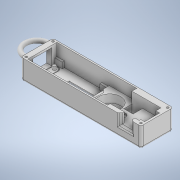
# Autodesk Inventor part: RespiraCheck-Enclosure-Top
Saved by Autodesk Inventor 2022 (Build 260153000, 153)
## iProperties
Created: 2022-04-28
Part Number: RespiraCheck-Enclosure-Top
Material: Generic
Document SubType Name: Modeling
Designer: incep
Density: 1 g/cm^3
Appearance: Default
Author: incep
## iProperties of the stored document RespiraCheck-Enclosure-Top_3DPrint.ipt
Created: 2022-04-28
Part Number: RespiraCheck-Enclosure-Top_3DPrint
Material: Generic
Document SubType Name: Modeling
Designer: incep
Density: 1 g/cm^3
Appearance: Default
Author: incep
Autodesk Inventor part; units mm, degrees
ref_plane "YZ Plane" through (0, 0, 0) normal (1, 0, 0) x (0, 1, 0)
ref_plane "XZ Plane" through (0, 0, 0) normal (0, 1, 0) x (-1, 0, 0)
sketch "Sketch1" plane through (0, 0, 0) normal (0, 1, 0) x (-1, 0, 0)
  line L0 (56, 15) -> (-56, 15)
  line L1 (-56, 15) -> (-56, -15)
  line L2 (-56, -15) -> (56, -15)
  line L3 (56, -15) -> (56, 15)
  point P0 (0, 0)
  point P1 (-56, 0)
  point P2 (0, -15)
  dimension "d0" = 30
  dimension "d1" = 112
  constraints: 8 end point, 2 midpoint, 2 parallel, 1 horizontal, 1 horizontal alignment, 1 perpendicular, 1 vertical alignment
  measures "d0" distance of L2.end L0.start
  measures "d1" distance of L1.end L2.end
extrude "Extrusion1" add sketch "Sketch1" along normal blind 19
sketch "Sketch2" plane through (0, 19, 0) normal (0, 1, 0) x (1, 0, 0)
  circle A0 centre (-53.5, 12.5) radius 2.5 construction
  line L0 (56, 15) -> (-56, 15) construction
  line L1 (-56, 15) -> (-56, -15) construction
  circle A1 centre (-53.5, -12.5) radius 2.5 construction
  circle A2 centre (53.5, 12.5) radius 2.5 construction
  circle A3 centre (53.5, -12.5) radius 2.5 construction
  line L2 (-56, -15) -> (56, -15) construction
  line L3 (56, -15) -> (56, 15) construction
  line L4 (-51, 13.6) -> (-2, 13.6)
  line L5 (-2, -13.6) -> (-51, -13.6)
  line L6 (-51, -13.6) -> (-51, 13.6)
  line L7 (-2, 8) -> (1, 8)
  line L8 (1, 8) -> (1, -8)
  line L9 (1, -8) -> (-2, -8)
  line L10 (-2, -8) -> (-2, 8) construction
  line L11 (-2, 8) -> (1, 5)
  line L12 (-2, -8) -> (1, -5)
  line L13 (-2, 13.6) -> (-2, 8)
  line L14 (-2, -8) -> (-2, -13.6)
  circle A4 centre (-53.5, 12.5) radius 1
  circle A5 centre (-53.5, -12.5) radius 1
  circle A6 centre (53.5, 12.5) radius 1
  circle A7 centre (53.5, -12.5) radius 1
  point P0 (0, 0)
  point P1 (-2, 0)
  point P2 (1, 0)
  point P3 (-51, 0)
  dimension "d4" = 5
  dimension "d5" = 5
  dimension "d6" = 5
  dimension "d7" = 5
  dimension "d8" = 27.2
  dimension "d10" = 3
  dimension "d11" = 16
  dimension "d14" = 49
  dimension "d15" = 45
  dimension "d16" = 45
  dimension "d64" = 2
  dimension "d65" = 2
  dimension "d66" = 2
  dimension "d67" = 2
  constraints: 22 end point, 9 tangent, 8 centre point, 5 parallel, 4 coincident, 3 perpendicular, 2 collinear, 2 horizontal, 2 horizontal alignment, 2 midpoint, 2 point on line
  measures "d4" diameter of A0
  measures "d5" diameter of A1
  measures "d6" diameter of A2
  measures "d7" diameter of A3
  measures "d8" distance of L5.end L4.start
  measures "d10" distance of L7.start L7.end
  measures "d11" distance of L7.end L8.end
  measures "d14" distance between parallel lines of L6 L13
  measures "d15" angle of L7 L11
  measures "d16" angle of L9 L12
  measures "d64" diameter of A4
  measures "d65" diameter of A5
  measures "d66" diameter of A6
  measures "d67" diameter of A7
extrude "Extrusion2" cut sketch "Sketch2" against normal blind 11.5 contours L4 L13 L11 L8 L12 L14 L5 L6 | A4 | A5 | A6 | A7
sketch "Sketch3" plane through (0, 7.5, 0) normal (0, 1, 0) x (1, 0, 0)
  line L0 (-2, 11.6) -> (-2, -11.6)
  line L1 (-51, -11.6) -> (-51, 11.6)
  line L2 (-51, -13.6) -> (-51, 13.6) projected
  line L3 (-2, 13.6) -> (-2, 8) projected
  line L4 (-9, -11.6) -> (-9, -13.6)
  line L5 (-9, -13.6) -> (-44, -13.6)
  line L6 (-44, -13.6) -> (-44, -11.6)
  line L7 (-2, -8) -> (-2, -13.6) projected
  line L8 (-2, -11.6) -> (-9, -11.6)
  line L9 (-44, -11.6) -> (-51, -11.6)
  line L10 (-51, 11.6) -> (-44, 11.6)
  line L11 (-9, 11.6) -> (-2, 11.6)
  line L12 (-51, 13.6) -> (-2, 13.6) projected
  line L13 (-9, 11.6) -> (-9, 13.6)
  line L14 (-9, 13.6) -> (-44, 13.6)
  line L15 (-44, 13.6) -> (-44, 11.6)
  line L16 (-2, -13.6) -> (-51, -13.6) projected
  point P0 (0, 0)
  point P1 (-2, 0)
  point P2 (-8.9823, 10)
  point P3 (-44, 13.6)
  dimension "d20" = 7
  dimension "d21" = 7
  dimension "d93" = 2
  dimension "d94" = 2
  dimension "d95" = 2
  constraints: 24 end point, 7 parallel, 4 collinear, 3 point on line, 2 horizontal, 2 perpendicular, 1 horizontal alignment, 1 midpoint, 1 vertical
  measures "d20" distance between parallel lines of L4 L7
  measures "d21" distance between parallel lines of L2 L6
  measures "d93" distance of L14.end L10.end
  measures "d94" distance of L11.start L13.end
  measures "d95" distance of L5.end L6.end
extrude "Extrusion3" cut sketch "Sketch3" against normal blind 5.5 contours L0 L8 L4 L5 L6 L9 L1 L10 L15 L12 L13 L11
sketch "Sketch4" plane through (0, 2, 0) normal (0, 1, 0) x (1, 0, 0)
  line L0 (-31, 5.1) -> (-7, 5.1)
  line L1 (-7, 5.1) -> (-7, -8.9)
  line L2 (-7, -8.9) -> (-31, -8.9)
  line L3 (-31, -8.9) -> (-31, 5.1)
  line L4 (-2, 8) -> (-2, -8) projected
  line L5 (-51, 13.6) -> (-2, 13.6) projected
  line L6 (-2, -13.6) -> (-51, -13.6) projected
  point P0 (0, 0)
  dimension "d24" = 5
  dimension "d25" = 8.5
  dimension "d26" = 4.7
  dimension "d27" = 24
  constraints: 8 end point, 2 parallel, 1 horizontal, 1 perpendicular
  measures "d24" distance between parallel lines of L4 L1
  measures "d25" distance between parallel lines of L0 L5
  measures "d26" distance between parallel lines of L6 L2
  measures "d27" distance between parallel lines of L3 L1
extrude "Extrusion4" cut sketch "Sketch4" against normal blind 2
sketch "Sketch5" plane through (0, 19, 0) normal (0, 1, 0) x (1, 0, 0)
  line L0 (-51, 13.6) -> (-2, 13.6) projected
  line L1 (-2, 13.6) -> (23.5, 13.6)
  line L2 (23.5, 13.6) -> (23.5, -13.6)
  line L3 (23.5, -13.6) -> (-2, -13.6)
  line L4 (-2, -13.6) -> (-2, 13.6)
  circle A0 centre (53.5, 12.5) radius 2.5 construction
  circle A1 centre (53.5, -12.5) radius 2.5 construction
  line L5 (-2, -13.6) -> (-51, -13.6) projected
  line L6 (1, 5) -> (1, -5) projected
  point P0 (0, 0)
  dimension "d43" = 22.5
  constraints: 8 end point, 2 parallel, 1 collinear, 1 horizontal, 1 perpendicular
  measures "d43" distance between parallel lines of L2 L6
extrude "Extrusion5" cut sketch "Sketch5" against normal blind 10.5
sketch "Sketch6" plane through (0, 8.5, 0) normal (0, 1, 0) x (1, 0, 0)
  circle A0 centre (12, 0) radius 10.1
  line L0 (1, -5) -> (1, 5) projected
  point P0 (0, 0)
  dimension "d32" = 20.2
  dimension "d33" = 11
  constraints: 1 centre point, 1 horizontal alignment
  measures "d32" diameter of A0
  measures "d33" distance from line of L0 A0.centre
extrude "Extrusion6" cut sketch "Sketch6" against normal blind 7.5
sketch "Sketch7" plane through (12, 1, 0) normal (0, 1, 0) x (1, 0, 0)
  circle A0 centre (0, 0) radius 10.1 projected
  circle A1 centre (0, 0) radius 6.5
  point P0 (-12, 0)
  dimension "d36" = 13
  constraints: 1 centre point, 1 coincident
  measures "d36" diameter of A1
extrude "Extrusion7" cut sketch "Sketch7" against normal blind 2 contours A1
sketch "Sketch8" plane through (0, 19, 0) normal (0, 1, 0) x (1, 0, 0)
  line L0 (23.5, 9.15) -> (50.6, 9.15)
  line L1 (50.6, 9.15) -> (50.6, -11.15)
  line L2 (50.6, -11.15) -> (23.5, -11.15)
  line L3 (23.5, -11.15) -> (23.5, 9.15)
  circle A0 centre (12, 0) radius 10.1 projected
  line L4 (23.5, -1) -> (50.6, -1) construction
  line L5 (23.5, 13.6) -> (23.5, -13.6) projected
  line L6 (50.6, 4.35) -> (54.1, 4.35)
  line L7 (54.1, 4.35) -> (54.1, -9.65)
  line L8 (54.1, -9.65) -> (50.6, -9.65)
  line L9 (50.6, -9.65) -> (50.6, 4.35)
  point P0 (0, 0)
  point P1 (50.6, 4.35)
  point P2 (50.6, -9.65)
  dimension "d39" = 20.3
  dimension "d42" = 1
  dimension "d46" = 27.1
  dimension "d47" = 14
  dimension "d48" = 3.5
  dimension "d49" = 1.5
  constraints: 18 end point, 4 parallel, 2 collinear, 2 horizontal, 2 midpoint, 2 perpendicular
  measures "d39" distance of L2.end L0.start
  measures "d42" vertical distance of L4.start A0.centre
  measures "d46" distance between parallel lines of L1 L3
  measures "d47" distance of L6.end L7.end
  measures "d48" distance of L6.start L6.end
  measures "d49" distance from line of L1.end L8
extrude "Extrusion8" cut sketch "Sketch8" against normal blind 9 contours L0 L1 L2 L3 | L6 L7 L8 L1
sketch "Sketch9" plane through (0, 10, 0) normal (0, 1, 0) x (1, 0, 0)
  line L0 (23.5, 9.15) -> (33.5, 9.15)
  line L1 (33.5, 9.15) -> (33.5, 0.15)
  line L2 (33.5, 0.15) -> (23.5, 0.15)
  line L3 (23.5, 0.15) -> (23.5, 9.15)
  line L4 (23.5, 9.15) -> (50.6, 9.15) projected
  line L5 (23.5, -11.15) -> (23.5, 9.15) projected
  point P0 (0, 0)
  dimension "d50" = 10
  dimension "d51" = 9
  constraints: 8 end point, 2 collinear, 2 parallel, 1 horizontal, 1 perpendicular
  measures "d50" distance of L1.end L2.end
  measures "d51" distance of L0.end L1.end
extrude "Extrusion9" cut sketch "Sketch9" against normal blind 10.5
sketch "Sketch10" plane through (50.6, 19, 11.15) normal (0, 0, -1) x (-1, 0, 0)
  line L0 (4, 0) -> (14, 0)
  line L1 (14, 0) -> (14, -9)
  line L2 (14, -9) -> (4, -9)
  line L3 (4, -9) -> (4, 0)
  line L4 (0, 0) -> (0, -9) projected
  line L5 (0, 0) -> (27.1, 0) projected
  line L6 (0, -9) -> (27.1, -9) projected
  point P0 (50.6, -19)
  dimension "d54" = 4
  dimension "d55" = 10
  constraints: 8 end point, 2 collinear, 2 parallel, 1 horizontal, 1 perpendicular
  measures "d54" distance between parallel lines of L4 L3
  measures "d55" distance between parallel lines of L1 L3
extrude "Extrusion10" cut sketch "Sketch10" against normal through all contours L0 L1 L2 L3
sketch "Sketch11" plane through (-56, 0, -15) normal (-1, 0, 0) x (0, 0, 1)
  line L0 (6, 17) -> (24, 17)
  line L1 (24, 17) -> (24, 2)
  line L2 (24, 2) -> (6, 2)
  line L3 (6, 2) -> (6, 17)
  line L4 (30, 0) -> (30, 19) projected
  line L5 (0, 0) -> (0, 19) projected
  line L6 (0, 0) -> (30, 0) projected
  line L7 (0, 19) -> (30, 19) projected
  point P0 (15, 0)
  dimension "d58" = 6
  dimension "d59" = 6
  dimension "d60" = 2
  dimension "d61" = 2
  constraints: 8 end point, 2 parallel, 1 horizontal, 1 perpendicular
  measures "d58" distance between parallel lines of L4 L1
  measures "d59" distance between parallel lines of L5 L3
  measures "d60" distance between parallel lines of L6 L2
  measures "d61" distance between parallel lines of L7 L0
extrude "Extrusion11" cut sketch "Sketch11" against normal up to surface (5 mm away) contours L0 L1 L2 L3
sketch "Sketch12" plane through (0, 0, 0) normal (0, -1, 0) x (1, 0, 0)
  line L0 (-39.2331, -12.5927) -> (-39.2331, 29.3378) construction
  line L1 (-39.2331, 29.3378) -> (-35.2988, 29.3378) construction
  line L2 (-35.2988, 29.3378) -> (-35.2988, -12.5927) construction
  line L3 (-35.2988, -12.5927) -> (-39.2331, -12.5927) construction
  line L4 (-36.3768, -10.4806) -> (-37.3923, -11.2247)
  spline S0 degree 2 poles (-37.3923, -11.2247) (-37.4874, -10.8555) (-37.9238, -10.5058) (-38.2455, -10.5058) knots 0 0 0 1 2 2 2
  spline S1 degree 2 poles (-38.2455, -10.5058) (-38.4554, -10.5058) (-38.8023, -10.654) (-38.9226, -10.7967) knots 0 0 0 1 2 2 2
  spline S2 degree 2 poles (-38.9226, -10.7967) (-39.0345, -10.9254) (-39.1268, -11.2723) (-39.1268, -11.5465) knots 0 0 0 1 2 2 2
  line L5 (-39.1268, -11.5465) -> (-39.1268, -12.3382)
  line L6 (-39.1268, -12.3382) -> (-36.3768, -12.3382)
  line L7 (-36.3768, -12.3382) -> (-36.3768, -11.829)
  line L8 (-36.3768, -11.829) -> (-37.4315, -11.829)
  line L9 (-37.4315, -11.829) -> (-36.3768, -11.11)
  line L10 (-36.3768, -11.11) -> (-36.3768, -10.4806)
  spline S3 degree 2 poles (-38.2316, -11.0205) (-38.0133, -11.0177) (-37.8119, -11.2863) (-37.8147, -11.58) knots 0 0 0 1 2 2 2
  line L11 (-37.8147, -11.58) -> (-37.8147, -11.829)
  line L12 (-37.8147, -11.829) -> (-38.64, -11.829)
  line L13 (-38.64, -11.829) -> (-38.64, -11.6024)
  spline S4 degree 2 poles (-38.64, -11.6024) (-38.64, -11.3646) (-38.5365, -11.11) (-38.3546, -11.0177) (-38.2316, -11.0205) knots 0 0 0 1 2 3 3 3
  spline S5 degree 2 poles (-37.3783, -8.1726) (-37.7, -8.1754) (-38.198, -8.4496) (-38.4833, -8.9279) (-38.4861, -9.2385) knots 0 0 0 1 2 3 3 3
  spline S6 degree 2 poles (-38.4861, -9.2385) (-38.4833, -9.5434) (-38.1952, -10.033) (-37.7084, -10.3211) (-37.4007, -10.3239) knots 0 0 0 1 2 3 3 3
  spline S7 degree 2 poles (-37.4007, -10.3239) (-37.0957, -10.3211) (-36.6146, -10.0274) (-36.332, -9.5266) (-36.3292, -9.2077) knots 0 0 0 1 2 3 3 3
  spline S8 degree 2 poles (-36.3292, -9.2077) (-36.3292, -8.9979) (-36.4803, -8.6006) (-36.774, -8.2985) (-36.9866, -8.2258) knots 0 0 0 1 2 3 3 3
  line L14 (-36.9866, -8.2258) -> (-36.9866, -8.7657)
  spline S9 degree 2 poles (-36.9866, -8.7657) (-36.8775, -8.858) (-36.7824, -9.0678) (-36.7824, -9.2189) knots 0 0 0 1 2 2 2
  spline S10 degree 2 poles (-36.7824, -9.2189) (-36.7852, -9.4427) (-37.0006, -9.742) (-37.1881, -9.7896) knots 0 0 0 1 2 2 2
  line L15 (-37.1881, -9.7896) -> (-37.1881, -8.1922)
  spline S11 degree 2 poles (-37.1881, -8.1922) (-37.2384, -8.181) (-37.3251, -8.1726) (-37.3783, -8.1726) knots 0 0 0 1 2 2 2
  line L16 (-37.6245, -8.6622) -> (-37.6245, -9.8036)
  spline S12 degree 2 poles (-37.6245, -9.8036) (-37.8231, -9.7448) (-38.0329, -9.4511) (-38.0329, -9.2301) knots 0 0 0 1 2 2 2
  spline S13 degree 2 poles (-38.0329, -9.2301) (-38.0329, -9.0007) (-37.8231, -8.7097) (-37.6245, -8.6622) knots 0 0 0 1 2 2 2
  spline S14 degree 2 poles (-37.0314, -6.4913) (-37.258, -6.4857) (-37.5378, -6.7458) (-37.6357, -7.0648) knots 0 0 0 1 2 2 2
  spline S15 degree 2 poles (-37.6357, -7.0648) (-37.686, -7.2298) (-37.7476, -7.3809) (-37.8063, -7.4173) (-37.8595, -7.4145) knots 0 0 0 1 2 3 3 3
  spline S16 degree 2 poles (-37.8595, -7.4145) (-37.935, -7.4117) (-38.0329, -7.3082) (-38.0329, -7.2242) knots 0 0 0 1 2 2 2
  spline S17 degree 2 poles (-38.0329, -7.2242) (-38.0329, -7.1459) (-37.949, -7.048) (-37.8707, -7.0312) knots 0 0 0 1 2 2 2
  line L17 (-37.8707, -7.0312) -> (-37.8707, -6.5472)
  spline S18 degree 2 poles (-37.8707, -6.5472) (-38.0637, -6.5584) (-38.3379, -6.7486) (-38.4861, -7.048) (-38.4861, -7.2242) knots 0 0 0 1 2 3 3 3
  spline S19 degree 2 poles (-38.4861, -7.2242) (-38.4805, -7.518) (-38.128, -7.9012) (-37.8595, -7.9096) knots 0 0 0 1 2 2 2
  spline S20 degree 2 poles (-37.8595, -7.9096) (-37.6357, -7.9124) (-37.3475, -7.6411) (-37.2468, -7.3361) knots 0 0 0 1 2 2 2
  spline S21 degree 2 poles (-37.2468, -7.3361) (-37.1937, -7.1739) (-37.1181, -7.0228) (-37.0426, -6.9836) (-36.9838, -6.9864) knots 0 0 0 1 2 3 3 3
  spline S22 degree 2 poles (-36.9838, -6.9864) (-36.8943, -6.9892) (-36.7852, -7.1123) (-36.7824, -7.2102) knots 0 0 0 1 2 2 2
  spline S23 degree 2 poles (-36.7824, -7.2102) (-36.7824, -7.3165) (-36.8999, -7.4508) (-37.0314, -7.4844) knots 0 0 0 1 2 2 2
  line L18 (-37.0314, -7.4844) -> (-37.0314, -7.9852)
  spline S24 degree 2 poles (-37.0314, -7.9852) (-36.6733, -7.9404) (-36.3292, -7.5403) (-36.3292, -7.227) knots 0 0 0 1 2 2 2
  spline S25 degree 2 poles (-36.3292, -7.227) (-36.332, -7.02) (-36.5167, -6.6871) (-36.8328, -6.4941) (-37.0314, -6.4913) knots 0 0 0 1 2 3 3 3
  spline S26 degree 2 poles (-37.4147, -4.0602) (-37.728, -4.063) (-38.2092, -4.326) (-38.4833, -4.7876) (-38.4861, -5.0869) knots 0 0 0 1 2 3 3 3
  spline S27 degree 2 poles (-38.4861, -5.0869) (-38.4861, -5.2967) (-38.3351, -5.6436) (-38.1952, -5.7639) knots 0 0 0 1 2 2 2
  line L19 (-38.1952, -5.7639) -> (-38.4386, -5.7639)
  line L20 (-38.4386, -5.7639) -> (-38.4386, -6.2171)
  line L21 (-38.4386, -6.2171) -> (-35.6886, -6.2171)
  line L22 (-35.6886, -6.2171) -> (-35.6886, -5.7219)
  line L23 (-35.6886, -5.7219) -> (-36.5698, -5.7219)
  spline S28 degree 2 poles (-36.5698, -5.7219) (-36.4467, -5.5849) (-36.3292, -5.2771) (-36.3292, -5.0897) knots 0 0 0 1 2 2 2
  spline S29 degree 2 poles (-36.3292, -5.0897) (-36.332, -4.7903) (-36.6118, -4.326) (-37.0985, -4.063) (-37.4147, -4.0602) knots 0 0 0 1 2 3 3 3
  spline S30 degree 2 poles (-37.4035, -4.5582) (-37.1349, -4.5637) (-36.788, -4.8911) (-36.7824, -5.1428) knots 0 0 0 1 2 2 2
  spline S31 degree 2 poles (-36.7824, -5.1428) (-36.788, -5.4086) (-37.1349, -5.7471) (-37.4119, -5.7527) knots 0 0 0 1 2 2 2
  spline S32 degree 2 poles (-37.4119, -5.7527) (-37.6832, -5.7471) (-38.0273, -5.4114) (-38.0329, -5.1484) knots 0 0 0 1 2 2 2
  spline S33 degree 2 poles (-38.0329, -5.1484) (-38.0273, -4.8939) (-37.6776, -4.5637) (-37.4035, -4.5582) knots 0 0 0 1 2 2 2
  line L24 (-36.3768, -3.2657) -> (-38.4386, -3.2657)
  line L25 (-38.4386, -3.2657) -> (-38.4386, -3.7608)
  line L26 (-38.4386, -3.7608) -> (-36.3768, -3.7608)
  line L27 (-36.3768, -3.7608) -> (-36.3768, -3.2657)
  line L28 (-38.7351, -3.2629) -> (-39.2303, -3.2629)
  line L29 (-39.2303, -3.2629) -> (-39.2303, -3.758)
  line L30 (-39.2303, -3.758) -> (-38.7351, -3.758)
  line L31 (-38.7351, -3.758) -> (-38.7351, -3.2629)
  line L32 (-38.0105, -1.9312) -> (-38.4861, -1.9312)
  line L33 (-38.4861, -1.9312) -> (-38.4861, -1.9676)
  spline S34 degree 2 poles (-38.4861, -1.9676) (-38.4889, -2.1215) (-38.377, -2.3201) (-38.2372, -2.4152) knots 0 0 0 1 2 2 2
  line L34 (-38.2372, -2.4152) -> (-38.4386, -2.4152)
  line L35 (-38.4386, -2.4152) -> (-38.4386, -2.8684)
  line L36 (-38.4386, -2.8684) -> (-36.3768, -2.8684)
  line L37 (-36.3768, -2.8684) -> (-36.3768, -2.3733)
  line L38 (-36.3768, -2.3733) -> (-37.5238, -2.3733)
  spline S35 degree 2 poles (-37.5238, -2.3733) (-37.7616, -2.3733) (-38.005, -2.155) (-38.0105, -1.9312) knots 0 0 0 1 2 2 2
  line L39 (-36.3768, 0.4103) -> (-38.4386, 0.4103)
  line L40 (-38.4386, 0.4103) -> (-38.4386, -0.0457)
  line L41 (-38.4386, -0.0457) -> (-38.1616, -0.0457)
  spline S36 degree 2 poles (-38.1616, -0.0457) (-38.3323, -0.1716) (-38.4861, -0.4961) (-38.4861, -0.7171) knots 0 0 0 1 2 2 2
  spline S37 degree 2 poles (-38.4861, -0.7171) (-38.4833, -1.0248) (-38.2064, -1.4948) (-37.7168, -1.7634) (-37.4007, -1.7662) knots 0 0 0 1 2 3 3 3
  spline S38 degree 2 poles (-37.4007, -1.7662) (-37.0874, -1.7634) (-36.6062, -1.4976) (-36.332, -1.0332) (-36.3292, -0.7283) knots 0 0 0 1 2 3 3 3
  spline S39 degree 2 poles (-36.3292, -0.7283) (-36.3292, -0.5129) (-36.4803, -0.1884) (-36.6453, -0.0457) knots 0 0 0 1 2 2 2
  line L42 (-36.6453, -0.0457) -> (-36.3768, -0.0457)
  line L43 (-36.3768, -0.0457) -> (-36.3768, 0.4103)
  spline S40 degree 2 poles (-37.3923, -0.0597) (-37.1293, -0.0625) (-36.788, -0.373) (-36.7824, -0.6584) knots 0 0 0 1 2 2 2
  spline S41 degree 2 poles (-36.7824, -0.6584) (-36.7852, -0.9325) (-37.1153, -1.2654) (-37.3895, -1.2682) knots 0 0 0 1 2 2 2
  spline S42 degree 2 poles (-37.3895, -1.2682) (-37.6748, -1.2626) (-38.0273, -0.9353) (-38.0329, -0.6667) knots 0 0 0 1 2 2 2
  spline S43 degree 2 poles (-38.0329, -0.6667) (-38.0273, -0.3954) (-37.6804, -0.0653) (-37.3923, -0.0597) knots 0 0 0 1 2 2 2
  line L44 (-37.1433, 3.4065) -> (-37.1433, 2.8078)
  spline S44 degree 2 poles (-37.1433, 2.8078) (-36.9699, 2.6428) (-36.8188, 2.321) (-36.8216, 2.128) knots 0 0 0 1 2 2 2
  spline S45 degree 2 poles (-36.8216, 2.128) (-36.8244, 1.8706) (-37.0762, 1.4538) (-37.4986, 1.2076) (-37.756, 1.2048) knots 0 0 0 1 2 3 3 3
  spline S46 degree 2 poles (-37.756, 1.2048) (-38.0189, 1.2076) (-38.4358, 1.4426) (-38.6792, 1.8511) (-38.682, 2.1168) knots 0 0 0 1 2 3 3 3
  spline S47 degree 2 poles (-38.682, 2.1168) (-38.6848, 2.3546) (-38.5169, 2.7015) (-38.3379, 2.8386) knots 0 0 0 1 2 2 2
  line L45 (-38.3379, 2.8386) -> (-38.3379, 3.4065)
  spline S48 degree 2 poles (-38.3379, 3.4065) (-38.7379, 3.2191) (-39.1715, 2.5337) (-39.1743, 2.1056) knots 0 0 0 1 2 2 2
  spline S49 degree 2 poles (-39.1743, 2.1056) (-39.1687, 1.7112) (-38.7911, 1.0733) (-38.1532, 0.6957) (-37.7616, 0.6901) knots 0 0 0 1 2 3 3 3
  spline S50 degree 2 poles (-37.7616, 0.6901) (-37.3615, 0.6957) (-36.7153, 1.0789) (-36.3348, 1.7308) (-36.3292, 2.1392) knots 0 0 0 1 2 3 3 3
  spline S51 degree 2 poles (-36.3292, 2.1392) (-36.3348, 2.5672) (-36.7628, 3.2386) (-37.1433, 3.4065) knots 0 0 0 1 2 2 2
  line L46 (-36.3768, 5.5075) -> (-37.5434, 5.5075)
  spline S52 degree 2 poles (-37.5434, 5.5075) (-38.0469, 5.5019) (-38.4945, 5.0738) (-38.4917, 4.699) knots 0 0 0 1 2 2 2
  spline S53 degree 2 poles (-38.4917, 4.699) (-38.4917, 4.5423) (-38.3966, 4.2849) (-38.2987, 4.1758) knots 0 0 0 1 2 2 2
  line L47 (-38.2987, 4.1758) -> (-39.1268, 4.1758)
  line L48 (-39.1268, 4.1758) -> (-39.1268, 3.6807)
  line L49 (-39.1268, 3.6807) -> (-36.3768, 3.6807)
  line L50 (-36.3768, 3.6807) -> (-36.3768, 4.1758)
  line L51 (-36.3768, 4.1758) -> (-37.4231, 4.1758)
  spline S54 degree 2 poles (-37.4231, 4.1758) (-37.7588, 4.1758) (-38.0385, 4.3968) (-38.0329, 4.6094) knots 0 0 0 1 2 2 2
  spline S55 degree 2 poles (-38.0329, 4.6094) (-38.0357, 4.8277) (-37.7504, 5.0151) (-37.4315, 5.0123) knots 0 0 0 1 2 2 2
  line L52 (-37.4315, 5.0123) -> (-36.3768, 5.0123)
  line L53 (-36.3768, 5.0123) -> (-36.3768, 5.5075)
  spline S56 degree 2 poles (-37.3783, 7.9749) (-37.7, 7.9721) (-38.198, 7.698) (-38.4833, 7.2196) (-38.4861, 6.909) knots 0 0 0 1 2 3 3 3
  spline S57 degree 2 poles (-38.4861, 6.909) (-38.4833, 6.6041) (-38.1952, 6.1145) (-37.7084, 5.8264) (-37.4007, 5.8236) knots 0 0 0 1 2 3 3 3
  spline S58 degree 2 poles (-37.4007, 5.8236) (-37.0957, 5.8264) (-36.6146, 6.1201) (-36.332, 6.6209) (-36.3292, 6.9398) knots 0 0 0 1 2 3 3 3
  spline S59 degree 2 poles (-36.3292, 6.9398) (-36.3292, 7.1496) (-36.4803, 7.5469) (-36.774, 7.849) (-36.9866, 7.9218) knots 0 0 0 1 2 3 3 3
  line L54 (-36.9866, 7.9218) -> (-36.9866, 7.3818)
  spline S60 degree 2 poles (-36.9866, 7.3818) (-36.8775, 7.2895) (-36.7824, 7.0797) (-36.7824, 6.9286) knots 0 0 0 1 2 2 2
  spline S61 degree 2 poles (-36.7824, 6.9286) (-36.7852, 6.7048) (-37.0006, 6.4055) (-37.1881, 6.3579) knots 0 0 0 1 2 2 2
  line L55 (-37.1881, 6.3579) -> (-37.1881, 7.9553)
  spline S62 degree 2 poles (-37.1881, 7.9553) (-37.2384, 7.9665) (-37.3251, 7.9749) (-37.3783, 7.9749) knots 0 0 0 1 2 2 2
  line L56 (-37.6245, 7.4853) -> (-37.6245, 6.3439)
  spline S63 degree 2 poles (-37.6245, 6.3439) (-37.8231, 6.4027) (-38.0329, 6.6964) (-38.0329, 6.9174) knots 0 0 0 1 2 2 2
  spline S64 degree 2 poles (-38.0329, 6.9174) (-38.0329, 7.1468) (-37.8231, 7.4378) (-37.6245, 7.4853) knots 0 0 0 1 2 2 2
  line L57 (-37.0538, 10.3277) -> (-37.0538, 9.7709)
  spline S65 degree 2 poles (-37.0538, 9.7709) (-36.9111, 9.6786) (-36.7824, 9.452) (-36.7824, 9.301) knots 0 0 0 1 2 2 2
  spline S66 degree 2 poles (-36.7824, 9.301) (-36.788, 9.038) (-37.1349, 8.7079) (-37.4119, 8.7023) knots 0 0 0 1 2 2 2
  spline S67 degree 2 poles (-37.4119, 8.7023) (-37.686, 8.7079) (-38.0273, 9.0296) (-38.0329, 9.2898) knots 0 0 0 1 2 2 2
  spline S68 degree 2 poles (-38.0329, 9.2898) (-38.0329, 9.4576) (-37.8931, 9.6954) (-37.7504, 9.7709) knots 0 0 0 1 2 2 2
  line L58 (-37.7504, 9.7709) -> (-37.7504, 10.3277)
  spline S69 degree 2 poles (-37.7504, 10.3277) (-38.1057, 10.2018) (-38.4833, 9.6479) (-38.4861, 9.2898) knots 0 0 0 1 2 2 2
  spline S70 degree 2 poles (-38.4861, 9.2898) (-38.4833, 8.982) (-38.2008, 8.4925) (-37.714, 8.2071) (-37.4063, 8.2043) knots 0 0 0 1 2 3 3 3
  spline S71 degree 2 poles (-37.4063, 8.2043) (-37.1041, 8.2071) (-36.6202, 8.5009) (-36.332, 8.996) (-36.3292, 9.3038) knots 0 0 0 1 2 3 3 3
  spline S72 degree 2 poles (-36.3292, 9.3038) (-36.332, 9.6674) (-36.7069, 10.1962) (-37.0538, 10.3277) knots 0 0 0 1 2 2 2
  line L59 (-36.3768, 12.5377) -> (-37.4287, 11.6817)
  line L60 (-37.4287, 11.6817) -> (-38.4386, 12.4202)
  line L61 (-38.4386, 12.4202) -> (-38.4386, 11.8271)
  line L62 (-38.4386, 11.8271) -> (-37.4678, 11.1697)
  line L63 (-37.4678, 11.1697) -> (-39.1268, 11.1697)
  line L64 (-39.1268, 11.1697) -> (-39.1268, 10.6746)
  line L65 (-39.1268, 10.6746) -> (-36.3768, 10.6746)
  line L66 (-36.3768, 10.6746) -> (-36.3768, 11.1697)
  line L67 (-36.3768, 11.1697) -> (-37.3419, 11.1697)
  line L68 (-37.3419, 11.1697) -> (-36.3768, 11.8719)
  line L69 (-36.3768, 11.8719) -> (-36.3768, 12.5377)
  point P0 (0, 0)
  constraints: 2 other
extrude "Extrusion12" cut sketch "Sketch12" against normal blind 1
chamfer "Chamfer1" distance 1 angle 45 9 edges at (-19, 0, 8.9) (-7, 0, 1.9) (-19, 0, -5.1) (-31, 0, 1.9) (5.5, 0, 0) (28.5, 0, -0.15) (23.5, 0, -4.65) (33.5, 0, -4.65) (28.5, 0, -9.15)
chamfer "Chamfer2" distance 2 angle 45 3 edges at (36.6, 14.5, 15) (41.6, 10, 15) (46.6, 14.5, 15)
fillet "Fillet1" radius 2 17 edges at (-19, 0, 9.8999) (-6.0001, 0, 1.9) (-19, 0, -6.0999) (-31.9999, 0, 1.9) (4.5001, 0, 0) (28.5, 0, 0.8499) (22.5001, 0, -4.65) (34.4999, 0, -4.65) (28.5, 0, -10.1499) (0, 0, -15) (56, 9.5, -15) (56, 0, 0) (0, 0, 15) (-56, 0, 0) (-56, 9.5, -15) (-56, 9.5, 15) (56, 9.5, 15)
sketch "Sketch13" plane through (-56, 17, -11.6) normal (-1, 0, 0) x (0, 0, 1)
  circle A0 centre (22.6, 0) radius 2
  line L0 (24.6, 2) -> (24.6, -15) projected
  line L1 (-1.4, 2) -> (24.6, 2) projected
  circle A1 centre (0.6, 0) radius 2
  line L2 (-1.4, -15) -> (-1.4, 2) projected
  point P0 (11.6, -17)
  dimension "d77" = 4
  dimension "d78" = 2
  dimension "d79" = 4
  dimension "d80" = 2
  constraints: 2 centre point, 2 tangent
  measures "d77" diameter of A0
  measures "d78" distance from line of L0 A0.centre
  measures "d79" diameter of A1
  measures "d80" distance from line of L2 A1.centre
ref_plane "Work Plane1" through (-56, 17, 11) normal (0, 1, 0) x (1, 0, 0)
sketch "Sketch14" plane through (-56, 17, 11) normal (0, 1, 0) x (1, 0, 0)
  line L0 (0, 2) -> (0, -2) projected
  line L1 (0, 20) -> (0, 2) projected
  arc A0 (0, 22) -> (0, 0) centre (0, 11) ccw
  line L2 (0, 24) -> (0, 20) construction
  line L3 (0, 0) -> (0, 22) construction
  point P0 (56, 11)
  constraints: 3 midpoint, 2 end point, 2 point on circle, 1 centre point
sweep "Sweep1" add profiles "Sketch13" path "Sketch14" path curves A0 contours A0
sketch "Sketch15" plane through (0, 10, 0) normal (0, 1, 0) x (1, 0, 0)
  circle A0 centre (29.5, -5.65) radius 3
  line L0 (23.5, -11.15) -> (23.5, 0.15) projected
  line L1 (36.6, -11.15) -> (23.5, -11.15) projected
  point P0 (0, 0)
  dimension "d83" = 6
  dimension "d84" = 6
  dimension "d85" = 5.5
  constraints: 1 centre point
  measures "d83" diameter of A0
  measures "d84" distance from line of A0.centre L0
  measures "d85" distance from line of L1 A0.centre
extrude "Extrusion13" cut sketch "Sketch15" against normal blind 1.5
sketch "Sketch16" plane through (0, 2, 0) normal (0, 1, 0) x (1, 0, 0)
  circle A0 centre (-47.5, 7.75) radius 1.5
  line L0 (-51, -13.6) -> (-51, 13.6) projected
  circle A1 centre (-47.5, -7.75) radius 1.5
  line L1 (-47.5, 7.75) -> (-47.5, -7.75) construction
  line L2 (-47.5, -7.75) -> (-47.5, 7.75) construction
  arc A2 (-51, -7.75) -> (-44, -7.75) centre (-47.5, -7.75) ccw
  arc A3 (-44, 7.75) -> (-51, 7.75) centre (-47.5, 7.75) ccw
  line L3 (-44.6, -7.75) -> (-44.6, 7.75)
  arc A4 (-44.6, 7.75) -> (-50.4, 7.75) centre (-47.5, 7.75) ccw
  line L4 (-50.4, 7.75) -> (-50.4, -7.75)
  arc A5 (-50.4, -7.75) -> (-44.6, -7.75) centre (-47.5, -7.75) ccw
  line L5 (-53, -1.1293) -> (-42.6, -1.1293)
  line L6 (-42.6, -1.1293) -> (-42.6, 1.1293)
  line L7 (-42.6, 1.1293) -> (-53, 1.1293)
  line L8 (-53, 1.1293) -> (-53, -1.1293)
  line L9 (-42, 1.7293) -> (-42, -1.7293)
  line L10 (-53.6, -1.7293) -> (-53.6, 1.7293)
  line L11 (-51, -1.7293) -> (-51, -7.75)
  line L12 (-51, 7.75) -> (-51, 1.7293)
  line L13 (-51, 1.1293) -> (-51, -1.1293)
  line L14 (-44, -7.75) -> (-44, -1.7293)
  line L15 (-44, -1.1293) -> (-44, 1.1293)
  line L16 (-44, 1.7293) -> (-44, 7.75)
  line L17 (-44, 1.7293) -> (-42, 1.7293)
  line L18 (-42, -1.7293) -> (-44, -1.7293)
  line L19 (-44.6, -1.7293) -> (-50.4, -1.7293)
  line L20 (-51, -1.7293) -> (-53.6, -1.7293)
  line L21 (-53.6, 1.7293) -> (-51, 1.7293)
  line L22 (-50.4, 1.7293) -> (-44.6, 1.7293)
  line L23 (-53, -1.1293) -> (-53.6, -1.1293)
  line L24 (-53, 1.1293) -> (-53.6, 1.1293)
  line L25 (-42.6, -1.1293) -> (-42, -1.1293)
  line L26 (-42.6, 1.1293) -> (-42, 1.1293)
  point P0 (0, 0)
  point P1 (-47.5, 0)
  point P2 (-47.5, 0)
  point P3 (-53, 0)
  point P4 (-50.4, 1.1293)
  point P5 (-44.6, 1.1293)
  point P6 (-51, 7.75)
  point P7 (-50.4, -1.1293)
  point P8 (-44.6, -1.1293)
  dimension "d88" = 3
  dimension "d90" = 3
  dimension "d91" = 15.5
  dimension "d92" = 3.5
  dimension "d96" = 0.6
  dimension "d98" = 2
  constraints: 54 end point, 22 parallel, 14 point on line, 12 tangent, 8 point on circle, 6 centre point, 6 perpendicular, 3 collinear, 3 midpoint, 2 horizontal alignment, 2 vertical, 1 horizontal
  measures "d88" diameter of A0
  measures "d90" diameter of A1
  measures "d91" distance of L1.start L1.end
  measures "d92" distance between parallel lines of L0 L1
  measures "d96" radial gap between concentric circles of A2 A5
  measures "d98" distance between parallel lines of L6 L3
extrude "Extrusion14" cut sketch "Sketch16" against normal up to surface (2 mm away) contours L0 L5 L4 A5 L3 L25 L9 L18 L14 A2 | L20 L10 L23 L5 L0 | L7 L24 L10 L21 L0 | L0 A3 L16 L17 L9 L26 L7 L3 A4 L4
extrude "Extrusion15" add sketch "Sketch16" along normal blind 3 contours A0 | A1
sketch "Sketch17" plane through (0, 0, 0) normal (0, -1, 0) x (1, 0, 0)
  line L0 (-48.5407, -9.6162) -> (-48.5407, 10.7144) construction
  line L1 (-48.5407, 10.7144) -> (-55.4282, 10.7144) construction
  line L2 (-55.4282, 10.7144) -> (-55.4282, -9.6162) construction
  line L3 (-55.4282, -9.6162) -> (-48.5407, -9.6162) construction
  line L4 (-46.5018, -7.5611) -> (-46.5018, -8.1721)
  line L5 (-46.5018, -8.1721) -> (-47.236, -8.728)
  line L6 (-47.236, -8.728) -> (-47.236, -8.9096)
  line L7 (-47.236, -8.9096) -> (-46.5018, -8.9096)
  line L8 (-46.5018, -8.9096) -> (-46.5018, -9.4088)
  line L9 (-46.5018, -9.4088) -> (-48.5018, -9.4088)
  line L10 (-48.5018, -9.4088) -> (-48.5018, -8.6049)
  spline S0 degree 2 poles (-48.5018, -8.6049) (-48.5018, -8.4379) (-48.4596, -8.1916) (-48.3948, -8.0862) knots 0 0 0 1 2 2 2
  spline S1 degree 2 poles (-48.3948, -8.0862) (-48.3267, -7.9793) (-48.1144, -7.8528) (-47.9524, -7.8528) knots 0 0 0 1 2 2 2
  spline S2 degree 2 poles (-47.9524, -7.8528) (-47.7238, -7.8528) (-47.437, -8.0603) (-47.3527, -8.2337) knots 0 0 0 1 2 2 2
  line L11 (-47.3527, -8.2337) -> (-46.5018, -7.5611)
  spline S3 degree 2 poles (-47.8891, -8.3682) (-47.9653, -8.3682) (-48.0739, -8.4266) (-48.1031, -8.493) knots 0 0 0 1 2 2 2
  spline S4 degree 2 poles (-48.1031, -8.493) (-48.1225, -8.54) (-48.1339, -8.6551) (-48.1339, -8.741) knots 0 0 0 1 2 2 2
  line L12 (-48.1339, -8.741) -> (-48.1339, -8.9096)
  line L13 (-48.1339, -8.9096) -> (-47.5958, -8.9096)
  line L14 (-47.5958, -8.9096) -> (-47.5958, -8.7653)
  spline S5 degree 2 poles (-47.5958, -8.7653) (-47.5958, -8.6616) (-47.6217, -8.5141) (-47.6622, -8.4639) knots 0 0 0 1 2 2 2
  spline S6 degree 2 poles (-47.6622, -8.4639) (-47.7011, -8.4152) (-47.8049, -8.3682) (-47.8891, -8.3682) knots 0 0 0 1 2 2 2
  line L15 (-46.5018, -7.412) -> (-48.5018, -7.412)
  line L16 (-48.5018, -7.412) -> (-48.5018, -6.0603)
  line L17 (-48.5018, -6.0603) -> (-48.1209, -6.0603)
  line L18 (-48.1209, -6.0603) -> (-48.1209, -6.9128)
  line L19 (-48.1209, -6.9128) -> (-47.7692, -6.9128)
  line L20 (-47.7692, -6.9128) -> (-47.7692, -6.1267)
  line L21 (-47.7692, -6.1267) -> (-47.3883, -6.1267)
  line L22 (-47.3883, -6.1267) -> (-47.3883, -6.9128)
  line L23 (-47.3883, -6.9128) -> (-46.8827, -6.9128)
  line L24 (-46.8827, -6.9128) -> (-46.8827, -6.0603)
  line L25 (-46.8827, -6.0603) -> (-46.5018, -6.0603)
  line L26 (-46.5018, -6.0603) -> (-46.5018, -7.412)
  spline S7 degree 2 poles (-46.4661, -5.1024) (-46.4661, -5.3326) (-46.5553, -5.6794) (-46.6201, -5.8285) knots 0 0 0 1 2 2 2
  line L27 (-46.6201, -5.8285) -> (-47.0966, -5.8285)
  line L28 (-47.0966, -5.8285) -> (-47.0966, -5.7831)
  spline S8 degree 2 poles (-47.0966, -5.7831) (-46.9686, -5.6324) (-46.8308, -5.271) (-46.8308, -5.1008) knots 0 0 0 1 2 2 2
  spline S9 degree 2 poles (-46.8308, -5.1008) (-46.8308, -5.057) (-46.8502, -4.916) (-46.8697, -4.8739) knots 0 0 0 1 2 2 2
  spline S10 degree 2 poles (-46.8697, -4.8739) (-46.8924, -4.822) (-46.975, -4.7491) (-47.0415, -4.7491) knots 0 0 0 1 2 2 2
  spline S11 degree 2 poles (-47.0415, -4.7491) (-47.1177, -4.7491) (-47.2117, -4.8674) (-47.2327, -4.9485) knots 0 0 0 1 2 2 2
  spline S12 degree 2 poles (-47.2327, -4.9485) (-47.2603, -5.0506) (-47.3073, -5.2823) (-47.343, -5.3844) knots 0 0 0 1 2 2 2
  spline S13 degree 2 poles (-47.343, -5.3844) (-47.424, -5.6162) (-47.7011, -5.8172) (-47.9086, -5.8172) knots 0 0 0 1 2 2 2
  spline S14 degree 2 poles (-47.9086, -5.8172) (-48.189, -5.8172) (-48.5374, -5.3423) (-48.5374, -4.9857) knots 0 0 0 1 2 2 2
  spline S15 degree 2 poles (-48.5374, -4.9857) (-48.5374, -4.8075) (-48.4645, -4.4541) (-48.4029, -4.3147) knots 0 0 0 1 2 2 2
  line L29 (-48.4029, -4.3147) -> (-47.9459, -4.3147)
  line L30 (-47.9459, -4.3147) -> (-47.9459, -4.3585)
  spline S16 degree 2 poles (-47.9459, -4.3585) (-48.0415, -4.4703) (-48.1728, -4.7912) (-48.1728, -4.9598) knots 0 0 0 1 2 2 2
  spline S17 degree 2 poles (-48.1728, -4.9598) (-48.1728, -5.0263) (-48.1533, -5.13) (-48.1274, -5.1883) knots 0 0 0 1 2 2 2
  spline S18 degree 2 poles (-48.1274, -5.1883) (-48.1063, -5.2353) (-48.022, -5.3034) (-47.9702, -5.3034) knots 0 0 0 1 2 2 2
  spline S19 degree 2 poles (-47.9702, -5.3034) (-47.8924, -5.3034) (-47.8032, -5.1948) (-47.7676, -5.0392) knots 0 0 0 1 2 2 2
  spline S20 degree 2 poles (-47.7676, -5.0392) (-47.7449, -4.9387) (-47.7011, -4.7523) (-47.6639, -4.6454) knots 0 0 0 1 2 2 2
  spline S21 degree 2 poles (-47.6639, -4.6454) (-47.5877, -4.4379) (-47.3349, -4.2353) (-47.1274, -4.2353) knots 0 0 0 1 2 2 2
  spline S22 degree 2 poles (-47.1274, -4.2353) (-46.8292, -4.2353) (-46.4661, -4.7037) (-46.4661, -5.1024) knots 0 0 0 1 2 2 2
  line L31 (-46.5018, -3.9776) -> (-48.5018, -3.9776)
  line L32 (-48.5018, -3.9776) -> (-48.5018, -2.6259)
  line L33 (-48.5018, -2.6259) -> (-48.1209, -2.6259)
  line L34 (-48.1209, -2.6259) -> (-48.1209, -3.4784)
  line L35 (-48.1209, -3.4784) -> (-47.7692, -3.4784)
  line L36 (-47.7692, -3.4784) -> (-47.7692, -2.6924)
  line L37 (-47.7692, -2.6924) -> (-47.3883, -2.6924)
  line L38 (-47.3883, -2.6924) -> (-47.3883, -3.4784)
  line L39 (-47.3883, -3.4784) -> (-46.8827, -3.4784)
  line L40 (-46.8827, -3.4784) -> (-46.8827, -2.6259)
  line L41 (-46.8827, -2.6259) -> (-46.5018, -2.6259)
  line L42 (-46.5018, -2.6259) -> (-46.5018, -3.9776)
  line L43 (-46.5018, -1.9015) -> (-48.1209, -1.9015)
  line L44 (-48.1209, -1.9015) -> (-48.1209, -2.493)
  line L45 (-48.1209, -2.493) -> (-48.5018, -2.493)
  line L46 (-48.5018, -2.493) -> (-48.5018, -0.8075)
  line L47 (-48.5018, -0.8075) -> (-48.1209, -0.8075)
  line L48 (-48.1209, -0.8075) -> (-48.1209, -1.399)
  line L49 (-48.1209, -1.399) -> (-46.5018, -1.399)
  line L50 (-46.5018, -1.399) -> (-46.5018, -1.9015)
  spline S23 degree 2 poles (-46.4629, 5.0937) (-46.4629, 4.6431) (-47.0075, 4.1147) (-47.5002, 4.1147) knots 0 0 0 1 2 2 2
  spline S24 degree 2 poles (-47.5002, 4.1147) (-47.975, 4.1147) (-48.5407, 4.6447) (-48.5407, 5.0953) knots 0 0 0 1 2 2 2
  spline S25 degree 2 poles (-48.5407, 5.0953) (-48.5407, 5.2136) (-48.5131, 5.4049) (-48.4904, 5.4924) knots 0 0 0 1 2 2 2
  spline S26 degree 2 poles (-48.4904, 5.4924) (-48.4694, 5.5605) (-48.3997, 5.7209) (-48.3737, 5.7712) knots 0 0 0 1 2 2 2
  line L51 (-48.3737, 5.7712) -> (-47.8973, 5.7712)
  line L52 (-47.8973, 5.7712) -> (-47.8973, 5.7209)
  spline S27 degree 2 poles (-47.8973, 5.7209) (-47.9297, 5.6836) (-48.0204, 5.5734) (-48.0626, 5.5037) knots 0 0 0 1 2 2 2
  spline S28 degree 2 poles (-48.0626, 5.5037) (-48.1063, 5.434) (-48.1663, 5.2671) (-48.1663, 5.1747) knots 0 0 0 1 2 2 2
  spline S29 degree 2 poles (-48.1663, 5.1747) (-48.1663, 5.0661) (-48.0982, 4.8862) (-48.0123, 4.8036) knots 0 0 0 1 2 2 2
  spline S30 degree 2 poles (-48.0123, 4.8036) (-47.9361, 4.729) (-47.6752, 4.6334) (-47.4985, 4.6334) knots 0 0 0 1 2 2 2
  spline S31 degree 2 poles (-47.4985, 4.6334) (-47.3122, 4.6334) (-47.0577, 4.7323) (-46.9799, 4.8133) knots 0 0 0 1 2 2 2
  spline S32 degree 2 poles (-46.9799, 4.8133) (-46.9037, 4.8911) (-46.8373, 5.0823) (-46.8373, 5.178) knots 0 0 0 1 2 2 2
  spline S33 degree 2 poles (-46.8373, 5.178) (-46.8373, 5.2768) (-46.9037, 5.4567) (-46.9443, 5.5183) knots 0 0 0 1 2 2 2
  spline S34 degree 2 poles (-46.9443, 5.5183) (-46.9848, 5.5864) (-47.0707, 5.6885) (-47.1047, 5.7258) knots 0 0 0 1 2 2 2
  line L53 (-47.1047, 5.7258) -> (-47.1047, 5.7712)
  line L54 (-47.1047, 5.7712) -> (-46.6347, 5.7712)
  spline S35 degree 2 poles (-46.6347, 5.7712) (-46.6088, 5.716) (-46.5439, 5.5718) (-46.5212, 5.494) knots 0 0 0 1 2 2 2
  spline S36 degree 2 poles (-46.5212, 5.494) (-46.4921, 5.4) (-46.4629, 5.2363) (-46.4629, 5.0937) knots 0 0 0 1 2 2 2
  line L55 (-46.5018, 5.8522) -> (-48.5018, 6.528)
  line L56 (-48.5018, 6.528) -> (-48.5018, 7.0759)
  line L57 (-48.5018, 7.0759) -> (-46.5018, 7.7517)
  line L58 (-46.5018, 7.7517) -> (-46.5018, 7.2347)
  line L59 (-46.5018, 7.2347) -> (-46.9102, 7.1099)
  line L60 (-46.9102, 7.1099) -> (-46.9102, 6.481)
  line L61 (-46.9102, 6.481) -> (-46.5018, 6.3546)
  line L62 (-46.5018, 6.3546) -> (-46.5018, 5.8522)
  line L63 (-47.2733, 6.9997) -> (-47.9345, 6.7955)
  line L64 (-47.9345, 6.7955) -> (-47.2733, 6.5896)
  line L65 (-47.2733, 6.5896) -> (-47.2733, 6.9997)
  line L66 (-46.5018, 9.2849) -> (-46.5018, 7.9511)
  line L67 (-46.5018, 7.9511) -> (-48.5018, 7.9511)
  line L68 (-48.5018, 7.9511) -> (-48.5018, 8.4535)
  line L69 (-48.5018, 8.4535) -> (-46.8827, 8.4535)
  line L70 (-46.8827, 8.4535) -> (-46.8827, 9.2849)
  line L71 (-46.8827, 9.2849) -> (-46.5018, 9.2849)
  point P0 (0, 0)
  constraints: 2 other
extrude "Extrusion16" cut sketch "Sketch17" against normal blind 1
fillet "Fillet2" radius 2 3 edges at (48.6, 13.5, 15) (41.6, 8, 15) (34.6, 13.5, 15)
body "Solid1"
